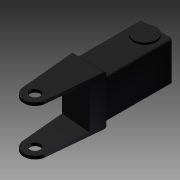
# Autodesk Inventor part: Bicep
Saved by Autodesk Inventor 2012 (Build 160160000, 160)
## iProperties
Created: 2013-03-08
Part Number: Bicep
Material: Default
Document SubType Name: Modeling
Designer: Andrew
Density: 1 g/cm^3
Author: Andrew
Autodesk Inventor part; units mm, degrees
ref_plane "YZ Plane" through (0, 0, 0) normal (1, 0, 0) x (0, 1, 0)
ref_plane "XZ Plane" through (0, 0, 0) normal (0, 1, 0) x (-1, 0, 0)
ref_plane "XY Plane" through (0, 0, 0) normal (0, 0, 1) x (1, 0, 0)
sketch "Sketch1" plane through (0, 0, 0) normal (0, 0, 1) x (1, 0, 0)
  circle A0 centre (0, 0) radius 11
  circle A1 centre (0, 106.7) radius 11
  line L0 (16, 106.7) -> (16, 53.35)
  line L1 (16, 107.3237) -> (16, 117.7)
  line L2 (16, 117.7) -> (-16, 117.7)
  line L3 (-16, 117.7) -> (-16, 53.35)
  line L4 (11, 0) -> (16, 53.35)
  line L5 (-11, 0) -> (-16, 53.35)
  line L6 (11, 0) -> (16, 53.35)
  line L7 (16, 53.35) -> (16, 117.7)
  line L8 (-16, 117.7) -> (-16, 53.35)
  line L9 (-11, 0) -> (-16, 53.35)
  line L10 (-16, 117.7) -> (16, 117.7)
  line L11 (16, 53.35) -> (-16, 53.35)
  dimension "d1" = 22
  dimension "d2" = 22
  dimension "d3" = 16
  dimension "d4" = 32
  constraints: 24 end point, 5 collinear, 3 parallel, 2 centre point, 2 point on circle, 1 coincident, 1 perpendicular
  measures "d1" diameter of A0
  measures "d2" diameter of A1
  measures "d3" distance of A1.centre L0.start
  measures "d4" distance of L1.end L2.end
extrude "Extrusion1" add sketch "Sketch1" along normal mid plane 48 contours A0 | A0 L5 L11 L4
extrude "Extrusion2" add sketch "Sketch1" along normal mid plane 38 contours A1 | L11 L3 L2 L1 L7 L0
extrude "Extrusion3" add sketch "Sketch1" along normal mid plane 42 contours A1
fillet "Fillet1" radius 2 8 edges at (16, 117.7, 0) (-16, 117.7, 0) (16, 85.525, 19) (-16, 85.525, 19) (-16, 85.525, -19) (16, 85.525, -19) (0, 53.35, -24) (0, 53.35, 24)
sketch "Sketch2" plane through (11, 0, 24) normal (0.9956369, -0.0933118, 0) x (0, 0, -1)
  ellipse E0 centre (2, 51.575) end of major axis (2, 53.5838) minor radius 2 (2, 53.5838) -> (0, 51.575) ccw projected
  line L0 (48, 0) -> (0, 0) projected
  line L1 (48, 0) -> (48, 51.575) projected
  line L2 (0, 0) -> (3, 0)
  line L3 (3, 0) -> (3, 38.5)
  line L4 (3, 38.5) -> (45, 38.5)
  line L5 (45, 38.5) -> (45, -15.2464)
  line L6 (45, -15.2464) -> (3, -15.2464)
  line L7 (3, -15.2464) -> (3, 0)
  point P0 (24, -1.0264)
  dimension "d12" = 3
  dimension "d13" = 38.5
  dimension "d14" = 42
  constraints: 12 end point, 3 perpendicular, 1 parallel, 1 point on line, 1 vertical, 1 other
  measures "d12" distance of L0.end L2.end
  measures "d13" distance of L2.end L3.end
  measures "d14" distance of L3.end L4.end
extrude "Extrusion4" cut sketch "Sketch2" along normal mid plane 100
sketch "Sketch3" plane through (0, 0, -24) normal (0, 0, -1) x (-1, 0, 0)
  arc A0 (-11, 0) -> (11, 0) centre (0, 0) ccw projected
  circle A1 centre (0, 0) radius 5
  dimension "d17" = 10
  constraints: 1 centre point, 1 coincident
  measures "d17" diameter of A1
extrude "Extrusion5" cut sketch "Sketch3" against normal through all
body "Solid1"
